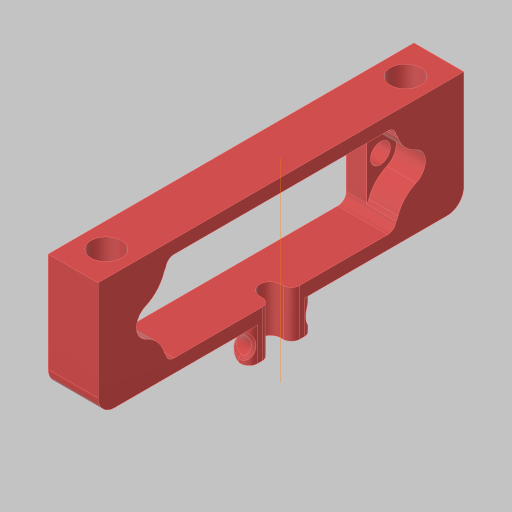
# Autodesk Inventor part: Spacer
Saved by Autodesk Inventor 2023.5 (Build 275446000, 446)
## iProperties
Created: 2025-02-08
Part Number: Spacer
Material: ABS Plastic
Document SubType Name: Modeling
Designer: slick
Density: 1.06 g/cm^3
Appearance: Smooth - Red
Author: slick
Autodesk Inventor part; units mm, degrees
ref_plane "YZ Plane" through (0, 0, 0) normal (1, 0, 0) x (0, 1, 0)
ref_plane "XZ Plane" through (0, 0, 0) normal (0, 1, 0) x (-1, 0, 0)
ref_plane "XY Plane" through (0, 0, 0) normal (0, 0, 1) x (1, 0, 0)
sketch "Sketch1" plane through (0, 0, 0) normal (1, 0, 0) x (0, 1, 0)
  line L0 (-11.1125, -34.925) -> (11.1125, -34.925)
  line L1 (11.1125, -34.925) -> (11.1125, 34.925)
  line L2 (11.1125, 34.925) -> (-11.1125, 34.925)
  line L3 (-11.1125, 34.925) -> (-11.1125, -34.925)
  line L4 (-11.1125, -34.925) -> (11.1125, 34.925) construction
  line L5 (11.1125, -34.925) -> (-11.1125, 34.925) construction
  point P0 (0, 0)
  dimension "d0" = 69.85
  dimension "d1" = 22.225
  constraints: 12 end point, 2 midpoint, 2 parallel, 1 horizontal, 1 perpendicular
  measures "d0" distance of L0.end L1.end
  measures "d1" distance between parallel lines of L3 L1
extrude "Extrusion1" add sketch "Sketch1" along normal blind 9.525
sketch "Sketch2" plane through (9.525, 0, 0) normal (1, 0, 0) x (0, 0, -1)
  line L0 (22, -8.5725) -> (-22, -8.5725)
  line L1 (-22, -8.5725) -> (-22, 8.5725)
  line L2 (-22, 8.5725) -> (22, 8.5725)
  line L3 (22, 8.5725) -> (22, -8.5725)
  line L4 (22, -8.5725) -> (-22, 8.5725) construction
  line L5 (-22, -8.5725) -> (22, 8.5725) construction
  circle A0 centre (-24.5942, 0) radius 3 construction
  circle A1 centre (24.5942, 0) radius 3 construction
  line L6 (-27.5942, 0) -> (27.5942, 0) construction
  arc A2 (-25.8022, 2.746) -> (-22, 8.5725) centre (-28.3653, 8.5725) ccw
  line L7 (0, 8.5725) -> (0, -8.5725) construction
  arc A3 (-22, -8.5725) -> (-25.8022, -2.746) centre (-28.3653, -8.5725) ccw
  arc A4 (22, 8.5725) -> (25.8022, 2.746) centre (28.3653, 8.5725) ccw
  arc A5 (25.8022, -2.746) -> (22, -8.5725) centre (28.3653, -8.5725) ccw
  arc A6 (-25.8022, 2.746) -> (-25.8022, -2.746) centre (-24.5942, 0) ccw
  arc A7 (25.8022, -2.746) -> (25.8022, 2.746) centre (24.5942, 0) ccw
  point P0 (0, 0)
  point P1 (0, 0)
  dimension "d4" = 44
  dimension "d5" = 17.145
  dimension "d7" = 6
  dimension "d20" = 49.1884
  constraints: 16 end point, 14 point on circle, 7 centre point, 6 coincident, 6 symmetric about line, 5 midpoint, 3 horizontal alignment, 2 horizontal, 2 parallel, 2 tangent, 1 perpendicular, 1 point on line, 6 other
  measures "d4" distance of L1.end L2.end
  measures "d5" distance of L0.end L1.end
  measures "d7" diameter of A0
  measures "d20" distance of A7.centre A0.centre
extrude "Extrusion2" cut sketch "Sketch2" against normal blind 5.6
hole "Hole1" at (9.525, 0, 24.5942) at (9.525, 0, -24.5942) direction (-1, 0, 0) diameter 3.81 end through all clearance for "Flat Head Machine Screw (82)" size "#6" standard "Ansi Unified Screw Threads"
fillet "Fillet1" radius 3.175 6 edges at (6.725, 8.5725, 22) (4.7625, -11.1125, 34.925) (6.725, -8.5725, 22) (6.725, -8.5725, -22) (4.7625, -11.1125, -34.925) (6.725, 8.5725, -22)
extrude "Extrusion4" cut sketch "Sketch2" against normal through all contours L0 L1 L2 L3
sketch "Sketch5" plane through (0, 11.1125, 28.575) normal (0, 1, 0) x (1, 0, 0)
  line L0 (4.7625, 0) -> (4.7625, 57.15) construction
  line L1 (0, 63.5) -> (0, -6.35) construction
  line L2 (0, 63.5) -> (9.525, 63.5) construction
  point P0 (0, 28.575)
  point P1 (4.7625, 28.575)
  point P2 (0, 28.575)
  point P3 (4.7625, 63.5)
  dimension "d26" = 57.15
  constraints: 3 midpoint, 2 end point, 2 vertical alignment, 1 horizontal alignment, 1 vertical
  measures "d26" distance of L0.start L0.end
hole "Hole2" at (4.7625, 11.1125, 28.575) at (4.7625, 11.1125, -28.575) direction (0, -1, 0) diameter 5.8 depth 7.62 tip angle 118
fillet "Fillet2" radius 1.5875 4 edges at (4.7625, -8.5725, -22) (4.7625, -8.5725, 22) (4.7625, 8.5725, -22) (4.7625, 8.5725, 22)
sketch "Sketch7" plane through (0, -11.1125, -31.75) normal (0, -1, 0) x (1, 0, 0)
  circle A0 centre (7.525, 31.75) radius 2
  line L0 (9.525, 63.5) -> (9.525, 0) construction
  line L1 (7.525, 33.75) -> (9.525, 33.75)
  line L2 (9.525, 52.1625) -> (9.525, 11.3375) construction
  line L3 (7.525, 29.75) -> (9.525, 29.75)
  line L4 (9.525, 29.75) -> (9.525, 33.75)
  point P0 (0, 31.75)
  point P1 (9.525, 31.75)
  dimension "d35" = 4
  dimension "d36" = 2
  constraints: 6 end point, 2 point on circle, 2 point on line, 2 tangent, 1 centre point, 1 collinear, 1 horizontal alignment, 1 midpoint, 1 parallel, 1 perpendicular
  measures "d35" diameter of A0
  measures "d36" distance from line of L0 A0.centre
extrude "Extrusion5" cut sketch "Sketch7" against normal up to surface (2.54 mm away)
fillet "Fillet3" radius 1.5875 2 edges at (9.525, -9.8425, -2) (9.525, -9.8425, 2)
sketch "Sketch8" plane through (0, -11.1125, -31.75) normal (0, -1, 0) x (1, 0, 0)
  line L0 (0, 0) -> (9.525, 0) construction
  line L1 (9.525, 28.1625) -> (9.525, 0) construction
  arc A0 (9.525, 28.1625) -> (7.9375, 29.75) centre (7.9375, 28.1625) ccw projected
  line L2 (7.525, 29.75) -> (7.9375, 29.75) projected
  arc A1 (7.525, 33.75) -> (7.525, 29.75) centre (7.525, 31.75) ccw projected
  line L3 (7.9375, 33.75) -> (7.525, 33.75) projected
  arc A2 (7.9375, 33.75) -> (9.525, 35.3375) centre (7.9375, 35.3375) ccw projected
  line L4 (9.525, 63.5) -> (9.525, 35.3375) construction
  line L5 (0, 63.5) -> (9.525, 63.5) construction
  line L6 (0, 0) -> (0, 63.5) construction
  line L7 (9.525, 52.1625) -> (9.525, 11.3375) construction
  arc A3 (9.525, 38.1) -> (9.525, 25.4) centre (9.525, 31.75) ccw
  line L8 (9.525, 11.3375) -> (9.525, 28.1625) construction
  line L9 (9.525, 25.4) -> (9.525, 28.1625)
  line L10 (9.525, 35.3375) -> (9.525, 52.1625) construction
  line L11 (9.525, 35.3375) -> (9.525, 38.1)
  point P0 (0, 31.75)
  dimension "d40" = 6.35
  constraints: 4 end point, 2 point on circle, 1 centre point, 1 collinear, 1 midpoint, 1 point on line, 1 vertical
  measures "d40" radius of A3
extrude "Extrusion6" add sketch "Sketch8" along normal blind 6.35
fillet "Fillet4" radius 1.5875 2 edges at (9.525, -14.2875, -6.35) (9.525, -14.2875, 6.35)
sketch "Sketch10" plane through (9.525, 0, 0) normal (1, 0, 0) x (0, 0, -1)
  line L0 (-4.4901, -17.4625) -> (-4.4901, -11.1125) construction
  line L1 (-3.5875, -17.4625) -> (-4.4901, -17.4625) construction
  line L2 (-3.5875, -8.5725) -> (-3.5875, -17.4625) construction
  line L3 (-3.5875, -8.5725) -> (-20.4125, -8.5725) construction
  arc A0 (-21.9861, -7.1949) -> (-20.4125, -8.5725) centre (-20.4125, -6.985) ccw construction
  arc A1 (-22.3628, -6.4541) -> (-21.9861, -7.1949) centre (-19.3688, -5.3975) ccw construction
  arc A2 (-22.3628, -6.4541) -> (-25.8022, -2.746) centre (-28.3653, -8.5725) ccw construction
  arc A3 (-25.8022, 2.746) -> (-25.8022, -2.746) centre (-24.5942, 0) ccw construction
  arc A4 (-25.8022, 2.746) -> (-22.3628, 6.4541) centre (-28.3653, 8.5725) ccw construction
  arc A5 (-21.9861, 7.1949) -> (-22.3628, 6.4541) centre (-19.3688, 5.3975) ccw construction
  arc A6 (-20.4125, 8.5725) -> (-21.9861, 7.1949) centre (-20.4125, 6.985) ccw construction
  line L4 (-20.4125, 8.5725) -> (20.4125, 8.5725) construction
  arc A7 (21.9861, 7.1949) -> (20.4125, 8.5725) centre (20.4125, 6.985) ccw construction
  arc A8 (22.3628, 6.4541) -> (21.9861, 7.1949) centre (19.3688, 5.3975) ccw construction
  arc A9 (22.3628, 6.4541) -> (25.8022, 2.746) centre (28.3653, 8.5725) ccw construction
  arc A10 (25.8022, -2.746) -> (25.8022, 2.746) centre (24.5942, 0) ccw construction
  arc A11 (25.8022, -2.746) -> (22.3628, -6.4541) centre (28.3653, -8.5725) ccw construction
  arc A12 (21.9861, -7.1949) -> (22.3628, -6.4541) centre (19.3688, -5.3975) ccw construction
  arc A13 (20.4125, -8.5725) -> (21.9861, -7.1949) centre (20.4125, -6.985) ccw construction
  line L5 (20.4125, -8.5725) -> (3.5875, -8.5725) construction
  line L6 (3.5875, -8.5725) -> (3.5875, -17.4625) construction
  line L7 (4.4901, -17.4625) -> (3.5875, -17.4625) construction
  line L8 (4.4901, -11.1125) -> (4.4901, -17.4625) construction
  line L9 (4.4901, -11.1125) -> (31.75, -11.1125) construction
  arc A14 (31.75, -11.1125) -> (34.925, -7.9375) centre (31.75, -7.9375) ccw construction
  line L10 (34.925, -7.9375) -> (34.925, 11.1125) construction
  line L11 (34.925, 11.1125) -> (-34.925, 11.1125) construction
  line L12 (-34.925, 11.1125) -> (-34.925, -7.9375) construction
  arc A15 (-34.925, -7.9375) -> (-31.75, -11.1125) centre (-31.75, -7.9375) ccw construction
  line L13 (-31.75, -11.1125) -> (-4.4901, -11.1125) construction
  line L14 (-6.0776, -11.1125) -> (-6.0776, -17.4625) construction
  arc A16 (-7.6651, -16.8443) -> (-7.6651, -11.7643) centre (-7.6651, -14.3043) ccw
  line L15 (0, 16.8275) -> (0, -23.1775) projected
  line L16 (-7.6651, -11.7643) -> (-7.6651, -16.8443)
  point P0 (0, 0)
  point P1 (-6.0776, -16.287)
  point P2 (-6.0776, -12.3215)
  point P3 (-7.6651, -14.3043)
  dimension "d48" = 2.54
  dimension "d49" = 1.5875
  constraints: 4 point on circle, 2 end point, 2 point on line, 1 centre point, 1 coincident, 1 midpoint, 1 vertical
  measures "d48" radius of A16
  measures "d49" distance from line of A16.centre L14
revolve "Revolution2" cut sketch "Sketch10" angle 360 about axis through (9.525, -11.1125, 0) along (0, -1, 0)
chamfer "Chamfer1" distance 0.4 angle 45 4 edges at (3.175, -16.4773, 0) (3.175, -12.1312, 0) (9.3932, -14.3043, 5.1234) (9.3932, -14.3043, -5.1234)
body "Solid1"
